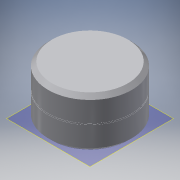
# Autodesk Inventor part: SweepV0.991_HEAD_Rev.1
Saved by Autodesk Inventor 2016 (Build 200138000, 138)
## iProperties
Created: 2018-03-01
Part Number: SweepV0.991_HEAD_Rev.1
Material: LCP Plastic
Document SubType Name: Modeling
Designer: emvanzant
Density: 1.626 g/cm^3
Appearance: Smooth - White
Author: emvanzant
Autodesk Inventor part; units mm, degrees
ref_plane "YZ Plane" through (0, 0, 0) normal (1, 0, 0) x (0, 1, 0)
ref_plane "XZ Plane" through (0, 0, 0) normal (0, 1, 0) x (-1, 0, 0)
sketch "Sketch1" plane through (0, 0, 0) normal (0, 1, 0) x (-1, 0, 0)
  circle A0 centre (0, 0) radius 32.5
  dimension "d0" = 65
  constraints: 1 centre point, 1 coincident
  measures "d0" diameter of A0
extrude "Extrusion1" add sketch "Sketch1" along normal blind 38.5
sketch "Sketch2" plane through (0, 0, 0) normal (0, -1, 0) x (1, 0, 0)
  circle A0 centre (0, 0) radius 25.5
  dimension "d3" = 51
  constraints: 1 centre point, 1 coincident
  measures "d3" diameter of A0
extrude "Extrusion2" add sketch "Sketch2" along normal blind 23.4
chamfer "Chamfer1" distance 3 angle 45 2 edges at (32.5, 38.5, 0) (32.5, 0, 0)
sketch "Sketch3" plane through (0, -23.4, 0) normal (0, -1, 0) x (1, 0, 0)
  line L0 (0, 0) -> (0, -10.5) construction
  circle A0 centre (0, 0) radius 25.5 projected
  line L1 (0, -10.5) -> (5.75, -10.5)
  line L2 (5.75, -10.5) -> (5.75, -24.8433)
  line L3 (0, -10.5) -> (-5.75, -10.5)
  line L4 (-5.75, -10.5) -> (-5.75, -24.8433)
  line L5 (5.75, -24.8433) -> (-5.75, -24.8433)
  line L6 (-15, 15) -> (15, 15) construction
  line L7 (15, 15) -> (15, -15) construction
  line L8 (15, -15) -> (-15, -15) construction
  line L9 (-15, -15) -> (-15, 15) construction
  line L10 (-15, 15) -> (15, -15) construction
  line L11 (15, 15) -> (-15, -15) construction
  line L12 (5.65, 5.65) -> (-5.65, 5.65) construction
  line L13 (-5.65, 5.65) -> (-5.65, -5.65) construction
  line L14 (-5.65, -5.65) -> (5.65, -5.65) construction
  line L15 (5.65, -5.65) -> (5.65, 5.65) construction
  line L16 (5.65, 5.65) -> (-5.65, -5.65) construction
  line L17 (-5.65, 5.65) -> (5.65, -5.65) construction
  dimension "d10" = 10.5
  dimension "d14" = 5.75
  dimension "d15" = 5.75
  dimension "d16" = 30
  dimension "d17" = 30
  dimension "d35" = 11.3
  dimension "d36" = 11.3
  constraints: 36 end point, 8 coincident, 4 horizontal, 4 midpoint, 4 parallel, 4 perpendicular, 2 point on circle, 1 vertical
  measures "d10" distance of L0.start L0.end
  measures "d14" distance of L0.end L1.end
  measures "d15" distance of L0.end L3.end
  measures "d16" distance of L7.end L8.end
  measures "d17" distance of L6.end L7.end
  measures "d35" distance of L14.end L13.end
  measures "d36" distance of L13.end L12.end
hole "Hole1" at (15, -23.4, -15) at (-15, -23.4, -15) at (15, -23.4, 15) at (-15, -23.4, 15) direction (0, 1, 0) diameter 2.5 depth 4 tip angle 118
thread "Thread1" size "M2.5x0.45" class "6H" standard "ANSI Metric M Profile" full length
thread "Thread2" size "M2.5x0.45" class "6H" standard "ANSI Metric M Profile" full length
thread "Thread3" size "M2.5x0.45" class "6H" standard "ANSI Metric M Profile" full length
thread "Thread4" size "M2.5x0.45" class "6H" standard "ANSI Metric M Profile" full length
extrude "Extrusion3" cut sketch "Sketch3" against normal blind 12 contours L5 A0 | L4 L3 L1 L2 L5
hole "Hole2" at (5.65, -23.4, 5.65) at (5.65, -23.4, -5.65) at (-5.65, -23.4, 5.65) at (-5.65, -23.4, -5.65) direction (0, 1, 0) diameter 2.1 depth 3 tip angle 118
thread "Thread5" size "M2.5x0.45" class "6H" standard "ANSI Metric M Profile" full length
thread "Thread6" size "M2.2x0.45" class "6H" standard "ANSI Metric M Profile" full length
thread "Thread7" size "M2.2x0.45" class "6H" standard "ANSI Metric M Profile" full length
thread "Thread8" size "M2.2x0.45" class "6H" standard "ANSI Metric M Profile" full length
ref_plane "Work Plane1" through (0, 0, -32.5) normal (0, 0, -1) x (-1, 0, 0)
sketch "Sketch4" plane through (0, 0, -32.5) normal (0, 0, -1) x (-1, 0, 0)
  line L0 (-25.5, -23.4) -> (25.5, -23.4) projected
  line L1 (-32.5, 3) -> (32.5, 3) projected
  line L2 (32.5, 35.5) -> (-32.5, 35.5) projected
  line L3 (0, -23.4) -> (0, 18.1) construction
  line L4 (32.5, 3) -> (32.5, 35.5) projected
  line L5 (-32.5, 3) -> (-32.5, 35.5) projected
  line L6 (32.5, 17.6) -> (32.5, 18.6)
  line L7 (-20, 18.1) -> (20, 18.1) construction
  line L8 (0, 18.1) -> (-15, 18.1)
  line L9 (0, 18.1) -> (15, 18.1)
  circle A0 centre (-15, 18.1) radius 6.35
  circle A1 centre (15, 18.1) radius 6.35
  point P0 (0, 0)
  point P1 (-5.75, -23.4)
  point P2 (5.75, -23.4)
  dimension "d52" = 41.5
  dimension "d53" = 1
  dimension "d54" = 20
  dimension "d56" = 15
  dimension "d57" = 15
  dimension "d58" = 12.7
  dimension "d59" = 12.7
  constraints: 12 end point, 2 centre point, 2 coincident, 2 midpoint, 2 point on line, 1 vertical
  measures "d52" distance of L3.start L3.end
  measures "d53" distance of L6.end L6.start
  measures "d54" distance of L3.end L7.end
  measures "d56" distance of L3.end L8.end
  measures "d57" distance of L3.end L9.end
  measures "d58" diameter of A0
  measures "d59" diameter of A1
extrude "Extrusion5" cut sketch "Sketch4" against normal blind 15 contours A0 | A1
sketch "Sketch6" plane through (0, 0, 0) normal (1, 0, 0) x (0, 1, 0)
  line L0 (3, 32.5) -> (35.5, 32.5) projected
  line L1 (35.5, 32.5) -> (19.25, 32.5)
  line L2 (19.25, 32.5) -> (19.75, 32.5)
  line L3 (19.25, 32.5) -> (18.75, 32.5)
  line L4 (18.875, 32.625) -> (18.625, 32.625)
  line L5 (18.625, 32.625) -> (18.625, 32.375)
  line L6 (18.625, 32.375) -> (18.875, 32.375)
  line L7 (18.875, 32.375) -> (18.875, 32.625)
  line L8 (18.875, 32.625) -> (18.625, 32.375) construction
  line L9 (18.625, 32.625) -> (18.875, 32.375) construction
  line L10 (19.875, 32.625) -> (19.625, 32.625)
  line L11 (19.625, 32.625) -> (19.625, 32.375)
  line L12 (19.625, 32.375) -> (19.875, 32.375)
  line L13 (19.875, 32.375) -> (19.875, 32.625)
  line L14 (19.875, 32.625) -> (19.625, 32.375) construction
  line L15 (19.625, 32.625) -> (19.875, 32.375) construction
  line L16 (-35.78, 0) -> (50.88, 0) projected
  point P0 (0, 0)
  dimension "d83" = 16.25
  dimension "d84" = 0.5
  dimension "d85" = 0.5
  dimension "d86" = 0.25
  dimension "d87" = 0.25
  dimension "d88" = 0.25
  dimension "d89" = 0.25
  constraints: 30 end point, 5 midpoint, 4 parallel, 2 horizontal, 2 perpendicular, 2 point on line
  measures "d83" distance of L0.end L1.end
  measures "d84" distance of L1.end L2.end
  measures "d85" distance of L1.end L3.end
  measures "d86" distance of L6.end L5.end
  measures "d87" distance of L5.end L4.end
  measures "d88" distance of L12.end L11.end
  measures "d89" distance of L11.end L10.end
revolve "Revolution4" cut sketch "Sketch6" angle 250 mid plane about axis through (0, -10, 0) along (0, 1, 0)
ref_plane "Work Plane2" through (0, 0, 0) normal (0, -1, 0) x (1, 0, 0)
split body "Split1" result two bodies by plane through (0, 0, 0) normal (0, -1, 0) first body at (-14.161, -15.6, -20.6026)
split "Split2" plane through (0, 0, 0) removes the side toward (0, -1, 0)
body "Solid2"
body "Solid3"
